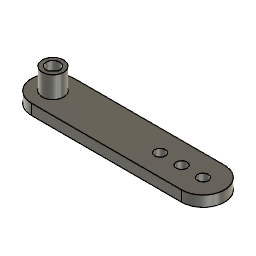
tige_capteur_axe_x_y (Autodesk Fusion 360 design; units mm, degrees)
Autodesk Fusion 360 part; units mm, degrees
sketch "Esquisse1" plane through (0, 0, 0) normal (0, 0, 1) x (1, 0, 0)
  circle A0 centre (0, 0) radius 10
  line L0 (0, 0) -> (70, 0)
  circle A1 centre (70, 0) radius 10
  line L1 (0, 10) -> (70, 10)
  line L2 (70, -10) -> (0, -10)
  constraint coincident A0.centre L0.start
  constraint horizontal L0
  constraint coincident L0.end A1.centre
  constraint coincident A0 L1.start
  constraint coincident A1 L1.end
  constraint tangent A1 L1
  constraint parallel L0 L1
  constraint coincident A1 L2.start
  constraint coincident A0 L2.end
  constraint tangent A0 L2
  constraint parallel L0 L2
extrude "Extrusion1" add sketch "Esquisse1" along normal blind 5
sketch "Esquisse2" plane through (0, 0, 5) normal (0, 0, 1) x (-1, 0, 0)
  arc A0 (0, -10) -> (0, 10) centre (0, 0) ccw
  line L0 (0, 10) -> (-70, 10)
  arc A1 (-70, 10) -> (-70, -10) centre (-70, 0) ccw
  line L1 (-70, -10) -> (0, -10)
  circle A2 centre (-70, 0) radius 2.5
  circle A3 centre (-60, 0) radius 2.5
  circle A4 centre (-50, 0) radius 2.5
  dimension "d3" = 5
  dimension "d4" = 5
  dimension "d5" = 5
  constraint concentric A1 A2
  measures "d3" diameter of A2
  measures "d4" diameter of A3
  measures "d5" diameter of A4
extrude "Extrusion2" cut sketch "Esquisse2" against normal blind 50 contours A2 | A3 | A4
sketch "Esquisse3" plane through (0, 0, 5) normal (0, 0, 1) x (-1, 0, 0)
  circle A0 centre (-50, 0) radius 2.5
  circle A1 centre (-60, 0) radius 2.5
  circle A2 centre (-70, 0) radius 2.5
  arc A3 (0, -10) -> (0, 10) centre (0, 0) ccw
  line L0 (0, 10) -> (-70, 10)
  arc A4 (-70, 10) -> (-70, -10) centre (-70, 0) ccw
  line L1 (-70, -10) -> (0, -10)
  circle A5 centre (0, 0) radius 3.5
  circle A6 centre (0, 0) radius 5
  dimension "d8" = 7
  constraint concentric A3 A5
  constraint concentric A5 A6
  measures "d8" diameter of A5
extrude "Extrusion3" add sketch "Esquisse3" along normal blind 12 contours A6
sketch "Esquisse4" plane through (0, 0, 5) normal (0, 0, 1) x (-1, 0, 0)
  circle A0 centre (0, 0) radius 3.5
  circle A1 centre (0, 0) radius 2
  line L0 (-2, 0) -> (-1, 0)
  line L1 (-1, 0) -> (-1, -1.7321)
  line L2 (-1, 1.7321) -> (-1, 0)
  dimension "d11" = 4
  constraint coincident A0.centre A1.centre
  constraint coincident A1 L0.start
  constraint horizontal L0
  constraint coincident A1 L1.end
  constraint perpendicular L0 L1
  constraint coincident A1 L2.start
  constraint perpendicular L0 L2
  measures "d11" diameter of A1
extrude "Extrusion4" add sketch "Esquisse4" along normal blind 6 contours A0 | A1 L0 L2 | A1 L0 L1
sketch "Esquisse5" plane through (0, 0, 17) normal (0, 0, 1) x (-1, 0, 0)
  circle A0 centre (0, 0) radius 3.5
  circle A1 centre (0, 0) radius 5
  line L0 (5, 0) -> (3.5, 0)
  line L1 (3.5, 0) -> (4, 0)
  line L2 (-5, 0) -> (-3.5, 0)
  line L3 (-3.5, 0) -> (-4, 0)
  circle A2 centre (0, 0) radius 4
  dimension "d14" = 0.5
  constraint coincident A1 L0.start
  constraint coincident A0 L0.end
  constraint horizontal L0
  constraint parallel L0 L1
  constraint coincident A1 L2.start
  constraint coincident A0 L2.end
  constraint horizontal L2
  constraint coincident L2 L3.end
  constraint coincident L3.end A2
  constraint coincident L1.end A2
  measures "d14" distance of L0.end L1.end
extrude "Extrusion5" cut sketch "Esquisse5" against normal blind 6 contours A0 L0 L1 L2 L3 A2 | A0 L0 L1 L2 L3 A2
extrude "Extrusion6" cut 1 faces at (2, 0, 11) along direction (0, 0, -1) blind 6
sketch "Esquisse6" plane through (0, 0, 5) normal (0, 0, 1) x (-1, 0, 0)
  circle A0 centre (0, 0) radius 4
  circle A1 centre (0, 0) radius 3.46
  dimension "d19" = 6.92
  constraint coincident A0.centre A1.centre
  measures "d19" diameter of A1
extrude "Extrusion7" add sketch "Esquisse6" along normal blind 12
sketch "Esquisse7" plane through (0, 0, 5) normal (0, 0, 1) x (-1, 0, 0)
  circle A0 centre (0, 0) radius 3.46
  circle A1 centre (0, 0) radius 1.975
  line L0 (1.5, 0) -> (1.975, 0)
  line L1 (1.975, 0) -> (-1.425, 0)
  line L2 (-1.425, 0) -> (-1.425, 1.3675)
  line L3 (-1.425, 0) -> (-1.425, -1.3675)
  dimension "d22" = 3.95
  dimension "d23" = 3.4
  constraint coincident A0.centre A1.centre
  constraint coincident A1 L0.end
  constraint horizontal L0
  constraint parallel L0 L1
  constraint coincident A1 L2.end
  constraint perpendicular L1 L2
  constraint coincident A1 L3.end
  constraint perpendicular L1 L3
  measures "d22" diameter of A1
  measures "d23" distance of L0.end L1.end
extrude "Extrusion8" add sketch "Esquisse7" along normal blind 6 contours A0 | A1 L2 L3
sketch "Esquisse8" plane through (0, 0, 17) normal (0, 0, 1) x (-1, 0, 0)
  circle A0 centre (0, 0) radius 3.46
  circle A1 centre (0, 0) radius 5
  circle A2 centre (0, 0) radius 3.5
  dimension "d26" = 7
  constraint coincident A0.centre A1.centre
  measures "d26" diameter of A2
extrude "Extrusion9" cut sketch "Esquisse8" against normal blind 6 contours A2
extrude "Extrusion10" cut 1 faces at (2.0648, 0.7997, 11) along direction (0, 0, -1) blind 6
sketch "Esquisse9" plane through (0, 0, 5) normal (0, 0, 1) x (-1, 0, 0)
  circle A0 centre (0, 0) radius 3.5
  circle A1 centre (0, 0) radius 2
  line L0 (2, 0) -> (-1.6, 0)
  line L1 (-1.6, 0) -> (-1.6, 1.2)
  line L2 (-1.6, 0) -> (-1.6, -1.2)
  dimension "d31" = 4
  dimension "d32" = 3.6
  constraint coincident A0.centre A1.centre
  constraint coincident A1 L0.start
  constraint horizontal L0
  constraint coincident A1 L1.end
  constraint perpendicular L0 L1
  constraint coincident A1 L2.end
  constraint perpendicular L0 L2
  measures "d31" diameter of A1
  measures "d32" distance of L0.start L0.end
extrude "Extrusion11" add sketch "Esquisse9" along normal blind 6 contours A0 | A1 L1 L2
sketch "Esquisse10" plane through (0, 0, 17) normal (0, 0, 1) x (-1, 0, 0)
  circle A0 centre (0, 0) radius 3.5
  circle A1 centre (0, 0) radius 5
  circle A2 centre (0, 0) radius 4
  dimension "d35" = 8
  constraint coincident A0.centre A1.centre
  measures "d35" diameter of A2
extrude "Extrusion12" cut sketch "Esquisse10" against normal blind 6 contours A2
sketch "Esquisse11" plane through (0, 0, 11) normal (0, 0, 1) x (-1, 0, 0)
  circle A0 centre (0, 0) radius 4
  line L0 (-1.6, -1.2) -> (-1.6, 1.2)
  arc A1 (-1.6, -1.2) -> (-1.6, 1.2) centre (0, 0) ccw
  circle A2 centre (0, 0) radius 2.05
  line L1 (0, 0) -> (-1.7, 0)
  line L2 (-1.7, 0) -> (-1.7, 1.1456)
  line L3 (-1.7, 0) -> (-1.7, -1.1456)
  dimension "d38" = 4.1
  dimension "d39" = 1.7
  constraint concentric A0 A2
  constraint coincident A0.centre A1.centre
  constraint perpendicular L0 L1
  constraint coincident A2 L2.end
  constraint perpendicular L1 L2
  constraint coincident A2 L3.end
  constraint perpendicular L1 L3
  measures "d38" diameter of A2
  measures "d39" distance of A0.centre L1.end
extrude "Extrusion13" cut sketch "Esquisse11" against normal blind 6 contours A2 L2 L3 picked at (-1.6333, 0.7819)
sketch "Esquisse12" plane through (0, 0, 5) normal (0, 0, 1) x (-1, 0, 0)
  arc A0 (0, -10) -> (0, 10) centre (0, 0) ccw
  line L0 (0, 10) -> (-70, 10)
  arc A1 (-70, 10) -> (-70, -10) centre (-70, 0) ccw
  line L1 (-70, -10) -> (0, -10)
  circle A2 centre (-70, 0) radius 2.5
  circle A3 centre (-60, 0) radius 2.5
  circle A4 centre (-50, 0) radius 2.5
  circle A5 centre (0, 0) radius 5
  circle A6 centre (0, 0) radius 6
  dimension "d42" = 12
  constraint concentric A0 A6
  measures "d42" diameter of A6
extrude "Extrusion14" add sketch "Esquisse12" along normal blind 12 contours A6
extrude "Extrusion15" cut 1 faces at (-5.2961, 0.4968, 17) along direction (0, 0, -1) blind 12
extrude "Extrusion16" add 1 faces at (2.4667, 0, 11) along direction (0, 0, -1) blind 6
extrude "Extrusion17" add 1 faces at (2.4667, 0, 11) along direction (0, 0, -1) blind 6
extrude "Extrusion18" add 1 faces at (2.4667, 0, 11) along direction (0, 0, -1) blind 6
delete_face "DeleteFace1" 1 faces at (-3.9801, 0.3983, 9)
sketch "Esquisse13" plane through (0, 0, 5) normal (0, 0, 1) x (-1, 0, 0)
  arc A0 (0, -10) -> (0, 10) centre (0, 0) ccw
  line L0 (0, 10) -> (-70, 10)
  arc A1 (-70, 10) -> (-70, -10) centre (-70, 0) ccw
  line L1 (-70, -10) -> (0, -10)
  circle A2 centre (-70, 0) radius 2.5
  circle A3 centre (-60, 0) radius 2.5
  circle A4 centre (-50, 0) radius 2.5
  circle A5 centre (0, 0) radius 3.2
  circle A6 centre (0, 0) radius 4.2
  line L2 (2, -2) -> (1, -1)
  line L3 (2, -2) -> (2.2627, -2.2627)
  line L4 (2.2627, -2.2627) -> (-1.9799, 1.9799)
  line L5 (-1.9799, 1.9799) -> (-0.8845, 3.0753)
  line L6 (-1.9799, 1.9799) -> (-3.0753, 0.8845)
  dimension "d53" = 6.4
  dimension "d54" = 8.4
  dimension "d55" = 6
  constraint coincident A0.centre A5.centre
  constraint concentric A5 A6
  constraint coincident A5 L3.end
  constraint parallel L2 L3
  constraint parallel L2 L4
  constraint coincident A5 L5.end
  constraint perpendicular L4 L5
  constraint coincident A5 L6.end
  constraint perpendicular L4 L6
  measures "d53" diameter of A5
  measures "d54" diameter of A6
  measures "d55" distance of L3.end L4.end
extrude "Extrusion19" add sketch "Esquisse13" along normal blind 10 contours A5 L5 L6 | A6
extrude "Extrusion20" cut 1 faces at (-0.9963, 0.0055, 5) along direction (0, 0, -1) blind 50
sketch "Esquisse14" plane through (0, 0, 5) normal (0, 0, 1) x (-1, 0, 0)
  circle A0 centre (-50, 0) radius 2.5
  circle A1 centre (-60, 0) radius 2.5
  circle A2 centre (-70, 0) radius 2.5
  arc A3 (0, -10) -> (0, 10) centre (0, 0) ccw
  line L0 (0, 10) -> (-70, 10)
  arc A4 (-70, 10) -> (-70, -10) centre (-70, 0) ccw
  line L1 (-70, -10) -> (0, -10)
  circle A5 centre (0, 0) radius 4.2
  circle A6 centre (0, 0) radius 5
  constraint coincident A3.centre A5.centre
extrude "Extrusion21" add sketch "Esquisse14" along normal blind 10 contours A6
